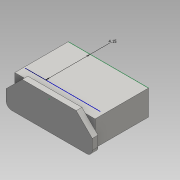
# Autodesk Inventor part: fciconnect-10118194
Saved by Autodesk Inventor 2016 (Build 200138000, 138)
## iProperties
Created: 2016-06-09
Part Number: fciconnect-10118194
Material: Generic
Document SubType Name: Modeling
Designer: admin
Density: 1 g/cm^3
Appearance: Default
Mass: 0.0996682 g
Surface Area: 1.5422 cm^2
Volume: 0.0996682 cm^3
Author: admin
Autodesk Inventor part; units mm, degrees
ref_plane "YZ Plane" through (0, 0, 0) normal (1, 0, 0) x (0, 1, 0)
ref_plane "XZ Plane" through (0, 0, 0) normal (0, 1, 0) x (-1, 0, 0)
ref_plane "XY Plane" through (0, 0, 0) normal (0, 0, 1) x (1, 0, 0)
sketch "Sketch1" plane through (0, 0, 0) normal (0, 1, 0) x (-1, 0, 0)
  line L0 (4.025, -0.9706) -> (4.025, 0)
  line L1 (2.525, 1.5) -> (-2.525, 1.5)
  line L2 (-4.025, 0) -> (-4.025, -0.9706)
  line L3 (-3.4956, -1.5) -> (3.4956, -1.5)
  arc A0 (3.4956, -1.5) -> (4.025, -0.9706) centre (3.4956, -0.9706) ccw
  arc A1 (-4.025, -0.9706) -> (-3.4956, -1.5) centre (-3.4956, -0.9706) ccw
  line L4 (4.025, 0) -> (2.525, 1.5)
  line L5 (-2.525, 1.5) -> (-4.025, 0)
  line L6 (0, -0.8604) -> (0, 0.9209) construction
  line L7 (1.4098, 0) -> (-0.8759, 0) construction
  point P0 (0, 0)
  dimension "d0" = 45
  dimension "d1" = 8.05
  dimension "d2" = 3
  constraints: 16 end point, 4 point on circle, 4 tangent, 3 point on line, 2 centre point, 2 parallel, 1 equal radius, 1 horizontal, 1 perpendicular, 1 vertical, 3 other
  measures "d0" angle of L1 L4
  measures "d1" distance between parallel lines of L2 L0
  measures "d2" distance between parallel lines of L1 L3
extrude "Extrusion1" add sketch "Sketch1" along normal blind 0.53
sketch "Sketch2" plane through (0, 0.53, 0) normal (0, 1, 0) x (1, 0, 0)
  line L0 (-3.75, 1.175) -> (3.75, 1.175)
  line L1 (3.75, 1.175) -> (3.75, -1.175)
  line L2 (3.75, -1.175) -> (-3.75, -1.175)
  line L3 (-3.75, -1.175) -> (-3.75, 1.175)
  point P0 (0, 0)
  point P1 (3.75, 0)
  point P2 (0, 1.175)
  dimension "d5" = 2.35
  dimension "d6" = 7.5
  constraints: 8 end point, 2 midpoint, 2 parallel, 1 horizontal, 1 horizontal alignment, 1 perpendicular, 1 vertical alignment
  measures "d5" distance between parallel lines of L2 L0
  measures "d6" distance of L0.start L0.end
extrude "Extrusion2" add sketch "Sketch2" along normal blind 5
sketch "Sketch3" plane through (2.85, 0.53, 1.175) normal (0, 0, 1) x (1, 0, 0)
  line L0 (-6.4765, 0.85) -> (0.5376, 0.85)
  line L1 (-6.6, 5) -> (0.9, 5) projected
  point P0 (-2.85, -0.53)
  dimension "d9" = 4.15
  constraints: 2 end point, 1 horizontal
  measures "d9" distance between parallel lines of L1 L0
body "Solid1"
